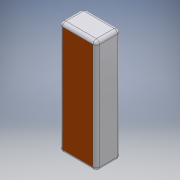
# Autodesk Inventor part: battery_vant_4500_4s
Saved by Autodesk Inventor 2016 (Build 200138000, 138)
## iProperties
Created: 2016-10-27
Part Number: battery_vant_4500_4s
Material: Generic
Document SubType Name: Modeling
Designer: Jakub
Density: 2.3183 g/cm^3
Appearance: Default
Mass: 390 g
Surface Area: 206.764 cm^2
Volume: 168.227 cm^3
Author: Jakub
Autodesk Inventor part; units mm, degrees
ref_plane "YZ Plane" through (0, 0, 0) normal (1, 0, 0) x (0, 1, 0)
ref_plane "XZ Plane" through (0, 0, 0) normal (0, 1, 0) x (-1, 0, 0)
ref_plane "XY Plane" through (0, 0, 0) normal (0, 0, 1) x (1, 0, 0)
sketch "Sketch1" plane through (0, 0, 0) normal (0, 0, 1) x (1, 0, 0)
  line L0 (-22, -14.5) -> (22, -14.5)
  line L1 (22, -14.5) -> (22, 14.5)
  line L2 (22, 14.5) -> (-22, 14.5)
  line L3 (-22, 14.5) -> (-22, -14.5)
  line L4 (-22, -14.5) -> (22, 14.5) construction
  line L5 (22, -14.5) -> (-22, 14.5) construction
  point P0 (0, 0)
  dimension "d0" = 44
  dimension "d1" = 29
  constraints: 12 end point, 2 midpoint, 2 parallel, 1 horizontal, 1 perpendicular
  measures "d0" distance of L2.end L1.end
  measures "d1" distance of L1.end L0.end
extrude "Extrusion1" add sketch "Sketch1" along normal blind 134
fillet "Fillet1" radius 4 12 edges at (0, 14.5, 134) (-22, 14.5, 67) (22, 14.5, 67) (0, -14.5, 134) (22, -14.5, 67) (-22, -14.5, 67) (0, 14.5, 0) (-22, 0, 0) (0, -14.5, 0) (22, 0, 0) (22, 0, 134) (-22, 0, 134)
body "Solid1"
